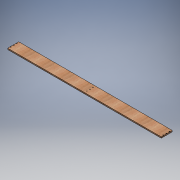
# Autodesk Inventor part: licht_200_back
Saved by Autodesk Inventor 2016 SP2 (Build 200236200, 236)
## iProperties
Created: 2018-01-11
Part Number: licht_200_back
Material: Spanplatte
Document SubType Name: Modeling
Designer: schueler
Density: 1 g/cm^3
Appearance: Birke - natur- poliert
Mass: 4605.71 g
Surface Area: 6469.23 cm^2
Volume: 4605.71 cm^3
Author: schueler
Autodesk Inventor part; units mm, degrees
ref_plane "YZ Plane" through (0, 0, 0) normal (1, 0, 0) x (0, 1, 0)
ref_plane "XZ Plane" through (0, 0, 0) normal (0, 1, 0) x (-1, 0, 0)
ref_plane "XY Plane" through (0, 0, 0) normal (0, 0, 1) x (1, 0, 0)
sketch "Skizze1" plane through (0, 0, 0) normal (0, 0, 1) x (1, 0, 0)
  line L0 (0, 0) -> (2000, 0)
  line L1 (2000, 0) -> (2000, 144)
  line L2 (2000, 144) -> (0, 144)
  line L3 (0, 144) -> (0, 0)
  line L4 (1000, 0) -> (1000, 144) construction
  line L5 (1992, 144) -> (1992, 0) construction
  line L6 (2000, 112) -> (0, 112) construction
  line L7 (2000, 32) -> (0, 32) construction
  circle A0 centre (1992, 112) radius 1.5
  circle A1 centre (1992, 32) radius 1.5
  line L8 (8, 144) -> (8, 0) construction
  circle A2 centre (8, 112) radius 1.5
  circle A3 centre (8, 72) radius 1.5
  circle A4 centre (8, 32) radius 1.5
  circle A5 centre (1992, 72) radius 1.5
  circle A6 centre (1000, 72) radius 1.5
  circle A7 centre (1000, 112) radius 1.5
  circle A8 centre (1000, 32) radius 1.5
  point P0 (2000, 72)
  dimension "d0" = 2000
  dimension "d1" = 144
  dimension "d20" = 8
  dimension "d21" = 40
  dimension "d22" = 40
  dimension "d23" = 3
  dimension "d24" = 3
  dimension "d25" = 8
  dimension "d26" = 3
  dimension "d27" = 3
  dimension "d28" = 3
  dimension "d29" = 3
  dimension "d30" = 3
  dimension "d31" = 3
  dimension "d32" = 3
  constraints: 18 end point, 16 point on line, 9 centre point, 8 midpoint, 4 perpendicular, 3 parallel, 1 horizontal
  measures "d0" distance of L2.end L1.end
  measures "d1" distance of L1.end L0.end
  measures "d20" distance of L1.end L5.start
  measures "d21" distance of L6.start point (2000, 72)
  measures "d22" distance of L7.start point (2000, 72)
  measures "d23" diameter of A0
  measures "d24" diameter of A1
  measures "d25" distance of L8.start L2.end
  measures "d26" diameter of A2
  measures "d27" diameter of A3
  measures "d28" diameter of A4
  measures "d29" diameter of A5
  measures "d30" diameter of A6
  measures "d31" diameter of A7
  measures "d32" diameter of A8
extrude "Extrusion1" add sketch "Skizze1" along normal blind 16
sketch "Skizze2" plane through (0, 0, 16) normal (0, 0, 1) x (1, 0, 0)
  circle A0 centre (1000, 72) radius 1.5 projected
  circle A1 centre (1992, 112) radius 1.5 projected
  circle A2 centre (1992, 72) radius 1.5 projected
  circle A3 centre (1992, 32) radius 1.5 projected
  circle A4 centre (8, 72) radius 1.5 projected
  circle A5 centre (8, 112) radius 1.5 projected
  circle A6 centre (8, 32) radius 1.5 projected
  circle A7 centre (1000, 32) radius 1.5 projected
  circle A8 centre (1000, 112) radius 1.5 projected
  point P0 (0, 0)
hole "Bohrung7" at (1000, 72, 16) at (1992, 112, 16) at (1992, 72, 16) at (1992, 32, 16) at (8, 72, 16) at (8, 32, 16) at (8, 112, 16) at (1000, 112, 16) at (1000, 32, 16) direction (0, 0, -1) diameter 3 depth 8 countersink diameter 8 countersink angle 90
sketch "Skizze3" plane through (0, 144, 0) normal (0, 1, 0) x (1, 0, 0)
  line L0 (0, 0) -> (2000, 0) construction
  line L1 (2000, 0) -> (2000, -16) construction
  line L2 (2000, -16) -> (0, -16) construction
  line L3 (0, -16) -> (0, 0) construction
  line L4 (0, 0) -> (0, -16) projected
  line L5 (0, -8) -> (2000, -8) construction
  line L6 (2000, 0) -> (2000, -16) projected
  line L7 (0, -16) -> (2000, -16) construction
  line L8 (1000, -16) -> (1000, 0) construction
  point P0 (750, -8)
  point P1 (250, -8)
  point P2 (1250, -8)
  point P3 (1750, -8)
  dimension "d120" = 250
  dimension "d121" = 250
  dimension "d122" = 250
  dimension "d123" = 250
  constraints: 12 end point, 4 midpoint, 4 point on line, 2 parallel, 1 horizontal, 1 perpendicular
  measures "d120" distance from line of L8 point (750, -8)
  measures "d121" distance from line of L3 point (250, -8)
  measures "d122" distance from line of L8 point (1250, -8)
  measures "d123" horizontal distance of L6.start point (1750, -8)
hole "Bohrung12" at (750, 144, 8) at (250, 144, 8) at (1250, 144, 8) at (1750, 144, 8) direction (0, -1, 0) diameter 3 depth 30 tip angle 118
